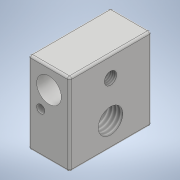
# Autodesk Inventor part: HotBlock
Saved by Autodesk Inventor 2020.2 (Build 242310000, 310)
## iProperties
Created: 2017-11-12
Part Number: HotBlock
Material: Ogólny
Document SubType Name: Modeling
Designer: Haras
Density: 1 g/cm^3
Appearance: Domyślna
Author: Haras
Autodesk Inventor part; units mm, degrees
ref_plane "YZ Plane" through (0, 0, 0) normal (1, 0, 0) x (0, 1, 0)
ref_plane "XZ Plane" through (0, 0, 0) normal (0, 1, 0) x (-1, 0, 0)
ref_plane "XY Plane" through (0, 0, 0) normal (0, 0, 1) x (1, 0, 0)
sketch "Szkic1" plane through (0, 0, 0) normal (1, 0, 0) x (0, 1, 0)
  line L0 (10, 10) -> (-10, 10)
  line L1 (-10, 10) -> (-10, -10)
  line L2 (-10, -10) -> (10, -10)
  line L3 (10, -10) -> (10, 10)
  line L4 (0, 0) -> (10, 0) construction
  line L5 (0, 0) -> (0, -10) construction
  dimension "d0" = 20
  dimension "d1" = 20
  constraints: 12 end point, 2 equal length, 2 midpoint, 2 vertical, 1 horizontal, 1 parallel
  measures "d0" distance of L2.end L0.start
  measures "d1" distance of L1.end L2.end
extrude "Wyciągnięcie proste1" add sketch "Szkic1" along normal blind 10
sketch "Szkic2" plane through (10, 0, 0) normal (1, 0, 0) x (0, 0, -1)
  line L0 (10, -10) -> (10, 10) projected
  point P0 (0, 0)
  point P1 (4, 0)
  dimension "d4" = 6
  constraints: 1 horizontal alignment
  measures "d4" distance from line of L0 point (4, 0)
hole "Otwór1" at (10, 0, -4) direction (-1, 0, 0) diameter 6 end through all
sketch "Szkic3" plane through (0, -10, -10) normal (0, -1, 0) x (1, 0, 0)
  line L0 (0, 20) -> (0, 0) projected
  line L1 (0, 20) -> (10, 20) projected
  point P0 (0, 10)
  point P1 (5, 15)
  dimension "d12" = 5
  dimension "d13" = 5
  measures "d12" distance from line of L0 point (5, 15)
  measures "d13" distance from line of L1 point (5, 15)
hole "Otwór2" at (5, -10, 5) direction (0, 1, 0) diameter 6 end through all
sketch "Szkic4" plane through (0, -10, -10) normal (0, -1, 0) x (1, 0, 0)
  line L0 (0, 20) -> (0, 0) projected
  point P0 (0, 10)
  point P1 (3, 10)
  point P2 (0, 10)
  dimension "d21" = 3
  constraints: 1 horizontal alignment, 1 midpoint
  measures "d21" distance of point (3, 10) point (0, 10)
hole "Otwór3" at (3, -10, 0) direction (0, 1, 0) diameter 2 depth 5 tip angle 118
sketch "Szkic5" plane through (10, 0, 0) normal (1, 0, 0) x (0, 0, -1)
  line L0 (-2, -10) -> (-8, -10) projected
  line L1 (-10, 10) -> (-10, -10) projected
  point P0 (0, 0)
  point P1 (-5, 0)
  dimension "d29" = 5
  constraints: 1 horizontal alignment
  measures "d29" distance from line of L1 point (-5, 0)
hole "Otwór4" at (10, 0, 5) direction (-1, 0, 0) diameter 3 depth 5 tip angle 118
thread "Gwint1" size "M3x0.5" class "6H" standard "ANSI Metric M Profile" full length
thread "Gwint2" size "M6x1" class "6H" standard "ANSI Metric M Profile" full length
fillet "Zaokrąglenie1" radius 0.5 12 edges at (0, 0, 10) (0, -10, 0) (5, -10, 10) (10, -10, 0) (10, 0, 10) (5, -10, -10) (0, 0, -10) (10, 0, -10) (5, 10, -10) (0, 10, 0) (10, 10, 0) (5, 10, 10)
